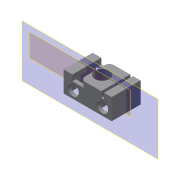
# Autodesk Inventor part: 04_OT_mic_slide_x
Saved by Autodesk Inventor 2019.4 (Build 234330000, 330)
## iProperties
Created: 2020-10-07
Part Number: 04_OT_mic_slide_x
Material: Generic
Document SubType Name: Modeling
Designer: diederichbenedict
Density: 1 g/cm^3
Appearance: Default
Author: diederichbenedict
Autodesk Inventor part; units mm, degrees
ref_plane "YZ Plane" through (0, 0, 0) normal (1, 0, 0) x (0, 1, 0)
ref_plane "XZ Plane" through (0, 0, 0) normal (0, 1, 0) x (-1, 0, 0)
ref_plane "XY Plane" through (0, 0, 0) normal (0, 0, 1) x (1, 0, 0)
ref_plane "Work Plane1" through (0, 0, -111.8) normal (0, 0, -1) x (-1, 0, 0)
sketch "Sketch1" plane through (0, 0, -111.8) normal (0, 0, -1) x (-1, 0, 0)
  circle A0 centre (-46.2034, -15) radius 3 projected
  circle A1 centre (-71.6034, -15) radius 3 projected
  line L0 (-79.6034, -22) -> (-38.2034, -22)
  line L1 (-38.2034, -22) -> (-38.2034, -4)
  line L2 (-38.2034, -4) -> (-79.6034, -4)
  line L3 (-79.6034, -4) -> (-79.6034, -22)
  circle A2 centre (-71.6034, -15) radius 5
  circle A3 centre (-46.2034, -15) radius 5
  point P0 (0, 0)
  dimension "d0" = 2
  dimension "d1" = 2
  dimension "d2" = 8
  dimension "d_4" = 8
  dimension "d4" = 11
  dimension "d5" = 7
  constraints: 8 end point, 2 centre point, 2 parallel, 1 horizontal, 1 perpendicular
  measures "d0" radial gap between concentric circles of A1 A2
  measures "d1" radial gap between concentric circles of A0 A3
  measures "d2" distance from line of L3 A1.centre
  measures "d_4" distance from line of L1 A0.centre
  measures "d4" distance from line of A0.centre L2
  measures "d5" distance from line of A1.centre L0
extrude "Extrusion1" add sketch "Sketch1" along normal mid plane 25 contours L3 L2 L1 L0
sketch "Sketch2" plane through (38.2034, -22, -124.3) normal (0, -1, 0) x (1, 0, 0)
  line L0 (28.4, 22.0118) -> (38.4, 22.0118) projected
  line L1 (38.4, 3.1118) -> (28.4, 3.1118) projected
  line L2 (36.4, 96.7206) -> (36.4, -103.2794)
  line L3 (30.4, 96.7206) -> (30.4, -103.2794)
  line L4 (39.55, 22) -> (27.25, 22)
  line L5 (27.25, 22) -> (27.25, 3)
  line L6 (27.25, 3) -> (39.55, 3)
  line L7 (39.55, 3) -> (39.55, 22)
  line L8 (0, 25) -> (41.4, 25) projected
  line L9 (41.4, 25) -> (0, 25) projected
  line L10 (20.7, 25) -> (20.7, 0)
  line L11 (41.4, 0) -> (0, 0) projected
  line L12 (13, 22.0118) -> (3, 22.0118)
  line L13 (3, 3.1118) -> (13, 3.1118)
  line L14 (1.85, 22) -> (14.15, 22)
  line L15 (14.15, 22) -> (14.15, 3)
  line L16 (14.15, 3) -> (1.85, 3)
  line L17 (1.85, 3) -> (1.85, 22)
  point P0 (-38.2034, 124.3)
  dimension "d8" = 19
  dimension "d9" = 12.3
  dimension "d10" = 3.15
  dimension "d11" = 3
  constraints: 26 end point, 8 symmetric about line, 2 midpoint, 2 parallel, 2 vertical, 1 horizontal, 1 perpendicular, 4 other
  measures "d8" distance between parallel lines of L6 L4
  measures "d9" distance between parallel lines of L7 L5
  measures "d10" distance between parallel lines of L7 L2
  measures "d11" distance between parallel lines of L8 L4
ref_plane "Work Plane2" through (0, 0, -111.8) normal (0, 0, 1) x (1, 0, 0)
extrude "Extrusion2" cut sketch "Sketch2" against normal blind 14 contours L4 L2 L1 L3 | L3 L6 L5 L4 | L4 L7 L6 L2 | L1 L2 L6 L3 | L14 L15 L16 L17
sketch "Sketch3" plane through (38.2034, -4, -124.3) normal (0, 1, 0) x (1, 0, 0)
  line L0 (41.4, -25) -> (41.4, 0) projected
  line L1 (0, 0) -> (41.4, 0) projected
  line L2 (0, -25) -> (0, 0) projected
  line L3 (41.4, -25) -> (0, -25) projected
  line L4 (34.7952, -26.219) -> (32.4952, -26.219)
  line L5 (32.4952, -26.219) -> (32.4952, 2.9805)
  line L6 (32.4952, 2.9805) -> (34.7952, 2.9805)
  line L7 (34.7952, 2.9805) -> (34.7952, -26.219)
  line L8 (14.4825, -27.0979) -> (7.5488, -27.0979)
  line L9 (7.5488, -27.0979) -> (7.5488, 2.9805)
  line L10 (7.5488, 2.9805) -> (14.4825, 2.9805)
  line L11 (14.4825, 2.9805) -> (14.4825, -27.0979)
  point P0 (-38.2034, -124.3)
  dimension "d14" = 2.3
  constraints: 16 end point, 4 parallel, 2 horizontal, 2 perpendicular
  measures "d14" distance of L5.end L6.end
extrude "Extrusion3" cut sketch "Sketch3" against normal blind 5 contours L7 L4 L5 L3 | L3 L5 L1 L7 | L1 L5 L6 L7 | L11 L8 L9 L3 | L3 L9 L1 L11 | L1 L9 L10 L11
fillet "Fillet1" radius 4 2 edges at (52.6859, -6.5, -124.3) (52.6859, -6.5, -99.3)
sketch "Sketch4" plane through (38.2034, -22, -124.3) normal (0, -1, 0) x (1, 0, 0)
  line L0 (27.25, 3) -> (27.25, 22) projected
  line L1 (27.25, 22) -> (39.55, 22) projected
  line L2 (39.55, 22) -> (39.55, 3) projected
  line L3 (39.55, 3) -> (27.25, 3) projected
  line L4 (1.85, 3) -> (1.85, 22) projected
  line L5 (1.85, 22) -> (14.15, 22) projected
  line L6 (14.15, 22) -> (14.15, 3) projected
  line L7 (14.15, 3) -> (1.85, 3) projected
  line L8 (0, 25) -> (0, 0) projected
  line L9 (41.4, 0) -> (0, 0) projected
  line L10 (41.4, 0) -> (41.4, 25) projected
  line L11 (0, 25) -> (41.4, 25) projected
  circle A0 centre (20.7, 12.5) radius 6.2
  point P0 (-38.2034, 124.3)
  dimension "d18" = 12.4
  constraints: 1 centre point
  measures "d18" diameter of A0
extrude "Extrusion4" cut sketch "Sketch4" against normal through all contours A0
sketch "Sketch5" plane through (38.2034, -22, -124.3) normal (0, -1, 0) x (1, 0, 0)
  circle A0 centre (20.7, 12.5) radius 6.2 projected
  line L0 (27.25, 3) -> (27.25, 22) projected
  line L1 (27.25, 22) -> (39.55, 22) projected
  line L2 (39.55, 22) -> (39.55, 3) projected
  line L3 (39.55, 3) -> (27.25, 3) projected
  line L4 (1.85, 3) -> (1.85, 22) projected
  line L5 (1.85, 22) -> (14.15, 22) projected
  line L6 (14.15, 22) -> (14.15, 3) projected
  line L7 (14.15, 3) -> (1.85, 3) projected
  line L8 (0, 25) -> (0, 0) projected
  line L9 (41.4, 0) -> (0, 0) projected
  line L10 (41.4, 0) -> (41.4, 25) projected
  line L11 (0, 25) -> (41.4, 25) projected
  circle A1 centre (16.15, 3) radius 1.45
  circle A2 centre (25.25, 22) radius 1.45
  circle A3 centre (20.7, 12.5) radius 8.6 construction
  point P0 (-38.2034, 124.3)
  dimension "d21" = 2.9
  dimension "d22" = 2.9
  dimension "d25" = 17.2
  dimension "d26" = 2
  dimension "d27" = 2
  constraints: 3 centre point, 3 coincident
  measures "d21" diameter of A1
  measures "d22" diameter of A2
  measures "d25" diameter of A3
  measures "d26" distance from line of A1.centre L6
  measures "d27" distance from line of A2.centre L0
extrude "Extrusion5" cut sketch "Sketch5" against normal blind 8 contours A1 | A2
equation "\"d2\" = d_4"
body "Solid1"
